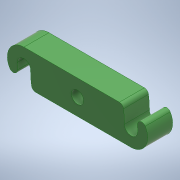
# Autodesk Inventor part: 071_0100_Base
Saved by Autodesk Inventor 2020 (Build 240168000, 168)
## iProperties
Created: 2018-07-06
Part Number: 071_0100_Base
Material: Generic
Document SubType Name: Modeling
Designer: deniz
Density: 1 g/cm^3
Appearance: Default
Author: deniz
Autodesk Inventor part; units mm, degrees
ref_plane "YZ Plane" through (0, 0, 0) normal (1, 0, 0) x (0, 1, 0)
ref_plane "XZ Plane" through (0, 0, 0) normal (0, 1, 0) x (-1, 0, 0)
ref_plane "XY Plane" through (0, 0, 0) normal (0, 0, 1) x (1, 0, 0)
sketch "Sketch1" plane through (0, 0, 0) normal (0, 1, 0) x (-1, 0, 0)
  line L0 (0, 0) -> (-51.4774, 0) construction
  line L1 (0, -8) -> (-51.4774, -8)
  line L2 (-51.4774, 8) -> (0, 8)
  arc A0 (0, -8) -> (0, 8) centre (0, 0) ccw
  arc A1 (-51.4774, 8) -> (-51.4774, -8) centre (-51.4774, 0) ccw
  circle A2 centre (0, 0) radius 2.6
  arc A3 (-50.8519, 8) -> (-51.4774, 0) centre (0, 0) ccw construction
  arc A4 (-54.0131, 8.4973) -> (-54.6774, 0) centre (0, 0) ccw
  arc A5 (-47.6908, 7.5027) -> (-48.2774, 0) centre (0, 0) ccw
  arc A6 (-47.6908, 7.5027) -> (-54.0131, 8.4973) centre (-50.8519, 8) ccw
  arc A7 (-54.6774, 0) -> (-48.2774, 0) centre (-51.4774, 0) ccw
  circle A8 centre (-25.7387, 0) radius 2.95
  circle A9 centre (-25.7387, 0) radius 6
  point P0 (-25.7387, 0)
  dimension "d8" = 51.4774
  dimension "d9" = 5.2
  dimension "d10" = 16
  dimension "d11" = 6.4
  dimension "d12" = 5.9
  dimension "d13" = 25.7387
  dimension "d18" = 12
  constraints: 14 point on circle, 10 centre point, 8 end point, 8 tangent, 3 coincident, 2 midpoint, 1 horizontal, 1 parallel, 1 point on line
  measures "d8" distance of L0.start L0.end
  measures "d9" diameter of A2
  measures "d10" distance between parallel lines of L1 L2
  measures "d11" diameter of A6
  measures "d12" diameter of A8
  measures "d13" distance of L0.start A8.centre
  measures "d18" diameter of A9
extrude "Extrusion3" add sketch "Sketch1" along normal blind 4 contours L1 A1 A4 A7 A5 A6 L2 A0 | A1 L2 A6 A5 A7 A4 | A9
extrude "Extrusion4" cut sketch "Sketch1" along normal blind 10 contours A4 A6 L2 A1 | A1 L2 A6 A5 A7 A4
pattern_circular "Circular Pattern1" count 2 over 360 about axis through (25.7387, 0, 0) along (0, 1, 0) of "Extrusion4"
extrude "Extrusion5" [suppressed]
move faces "Move1" translate (0, -8, 0) faces at (27.1324, 0, -6.3095)
fillet "Fillet2" radius 2 4 edges at (47.6519, -2, 8) (54.1552, -2, 7.5385) (-2.6778, -2, -7.5385) (3.8254, -2, -8)
equation "\"d8\" = d_clamp_total"
equation "\"d13\" = d_clamp_center"
equation "\"d_clamp_total\" = 51.477374"
equation "\"d_clamp_center\" = 25.738687"
body "Solid2"
